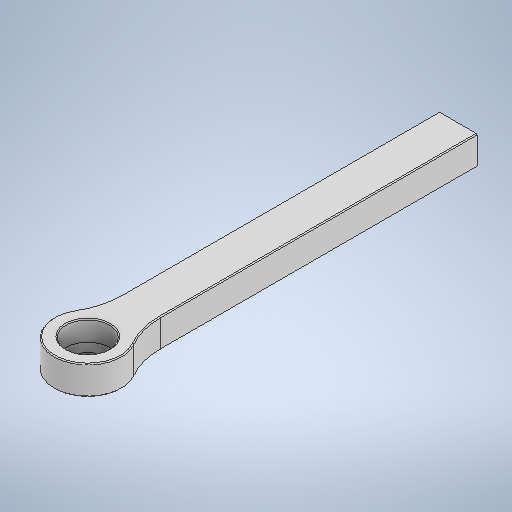
# Autodesk Inventor part: alternativeJoint2
Saved by Autodesk Inventor 2025.1 (Build 291241000, 241)
## iProperties
Created: 2024-11-07
Part Number: alternativeJoint2
Material: Generisch
Document SubType Name: Modeling
Designer: ZOMBULLI
Density: 1 g/cm^3
Appearance: Vorgabe
Author: ZOMBULLI
Autodesk Inventor part; units mm, degrees
ref_plane "YZ Plane" through (0, 0, 0) normal (1, 0, 0) x (0, 1, 0)
ref_plane "XZ Plane" through (0, 0, 0) normal (0, 1, 0) x (-1, 0, 0)
ref_plane "XY Plane" through (0, 0, 0) normal (0, 0, 1) x (1, 0, 0)
sketch "Skizze1" plane through (0, 0, 0) normal (0, 0, 1) x (1, 0, 0)
  line L0 (4, 77) -> (-4, 77)
  line L1 (-4, 77) -> (-4, 11.0905)
  line L2 (4, 11.0905) -> (4, 77)
  arc A0 (-6.0455, 3.5288) -> (6.0455, 3.5288) centre (0, 0) ccw
  arc A1 (4, 11.0905) -> (6.0455, 3.5288) centre (19, 11.0905) ccw
  arc A2 (-6.0455, 3.5288) -> (-4, 11.0905) centre (-19, 11.0905) ccw
  line L3 (0, -25.0931) -> (0, 22.9698)
  line L4 (0, 97.4186) -> (0, -45.5118) projected
  point P0 (0, 0)
  point P1 (0, 0)
  point P2 (-4, 5.7446)
  point P3 (4, 5.7446)
  dimension "d1" = 14
  dimension "d3" = 15
  dimension "d4" = 15
  dimension "d7" = 0
  dimension "d8" = 77
  dimension "d9" = 0
  dimension "d10" = 0
  dimension "d20" = 4
  dimension "d21" = 4
  constraints: 8 end point, 8 point on circle, 4 tangent, 3 centre point, 2 point on line, 1 horizontal, 1 parallel, 1 perpendicular
  measures "d1" diameter of A0
  measures "d3" radius of A1
  measures "d4" radius of A2
  measures "d7" distance of A0.centre point (0, 0)
  measures "d8" distance from line of point (0, 0) L0
  measures "d9" distance between parallel lines of L4 L3
  measures "d10" distance of point (0, 0) point (0, 0)
  measures "d20" distance between parallel lines of L4 L1
  measures "d21" distance between parallel lines of L4 L2
extrude "Extrusion1" add sketch "Skizze1" along normal blind 6
sketch "Skizze4" plane through (0, 0, 6) normal (0, 0, 1) x (1, 0, 0)
  circle A0 centre (0, 0) radius 4.5
  dimension "d22" = 9
  constraints: 1 centre point, 1 coincident
  measures "d22" diameter of A0
extrude "Extrusion2" cut sketch "Skizze4" against normal blind 4.2
fillet "Rundung1" radius 0.2 1 edges at (-4.5, 0, 6)
fillet "Rundung2" radius 0.2 10 edges at (4, 44.0453, 6) (0, -7, 6) (-4.5204, 7.1738, 6) (-4, 44.0453, 6) (4.5204, 7.1738, 6) (4, 44.0453, 0) (0, -7, 0) (-4.5204, 7.1738, 0) (-4, 44.0453, 0) (4.5204, 7.1738, 0)
sketch "Skizze5" plane through (0, 0, 0) normal (0, 0, -1) x (-1, 0, 0)
  circle A0 centre (0, 0) radius 1.75
  dimension "d27" = 3.5
  constraints: 1 centre point, 1 coincident
  measures "d27" diameter of A0
extrude "Extrusion3" cut sketch "Skizze5" against normal blind 4.2
fillet "Rundung3" radius 0.2 2 edges at (1.75, 0, 0) (1.75, 0, 1.8)
sketch "Skizze6" plane through (-3.8, 77, 0) normal (0, 1, 0) x (1, 0, 0)
  circle A0 centre (3.8, -3) radius 1.75
  line L0 (7.6, -6) -> (0, -6) projected
  line L1 (7.8, -0.2) -> (7.8, -5.8) projected
  point P0 (3.8, 0)
  dimension "d31" = 3.5
  dimension "d32" = 3
  dimension "d33" = 4
  constraints: 1 centre point
  measures "d31" diameter of A0
  measures "d32" distance from line of L0 A0.centre
  measures "d33" distance from line of A0.centre L1
extrude "Extrusion4" cut sketch "Skizze6" against normal blind 4
